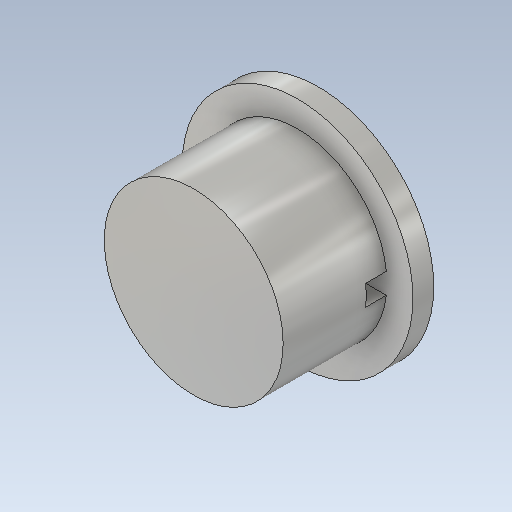
# Autodesk Inventor part: battery_endcap
Saved by Autodesk Inventor 2020 (Build 240168000, 168)
## iProperties
Created: 2017-11-26
Part Number: battery_endcap
Material: Generic
Document SubType Name: Modeling
Designer: stedrock
Density: 1 g/cm^3
Appearance: Default
Mass: 24.2995 g
Surface Area: 63.4336 cm^2
Volume: 24.2995 cm^3
Author: stedrock
Autodesk Inventor part; units mm, degrees
ref_plane "YZ Plane" through (0, 0, 0) normal (1, 0, 0) x (0, 1, 0)
ref_plane "XZ Plane" through (0, 0, 0) normal (0, 1, 0) x (-1, 0, 0)
ref_plane "XY Plane" through (0, 0, 0) normal (0, 0, 1) x (1, 0, 0)
sketch "Sketch1" plane through (0, 0, 0) normal (0, 0, 1) x (1, 0, 0)
  circle A0 centre (0, 0) radius 22.225
  circle A1 centre (0, 0) radius 17.225
  line L0 (-17.225, -2) -> (17.225, -2)
  line L1 (17.225, -2) -> (17.225, 2)
  line L2 (17.225, 2) -> (-17.225, 2)
  line L3 (-17.225, 2) -> (-17.225, -2)
  line L4 (-17.225, -2) -> (17.225, 2) construction
  line L5 (17.225, -2) -> (-17.225, 2) construction
  dimension "d0" = 44.45
  dimension "d1" = 34.45
  dimension "d2" = 4
  constraints: 12 end point, 2 centre point, 2 coincident, 2 midpoint, 2 parallel, 1 horizontal, 1 perpendicular, 1 tangent
  measures "d0" diameter of A0
  measures "d1" diameter of A1
  measures "d2" distance of L0.end L1.end
extrude "Extrusion1" add sketch "Sketch1" against normal blind 4 contours A0 | A1 L0 L2 | L1 L0 A1 | A1 L2 L1 | L2 A1 | A1 L0 | A1 L3 L2 | L0 L3 A1
extrude "Extrusion2" add sketch "Sketch1" along normal blind 20 contours A1 L0 L2 | L2 A1 | A1 L0
extrude "Extrusion3" cut sketch "Sketch1" along normal blind 4 contours A1 L0 L2 | L1 L0 A1 | A1 L2 L1 | A1 L3 L2 | L0 L3 A1
equation "\"d0\" = tube_ID"
equation "\"d3\" = sheet"
equation "\"d5\" = 5 * sheet"
equation "\"d7\" = sheet"
equation "\"tube_ID\" = 44.45"
equation "\"sheet\" = 4"
body "Solid1"
